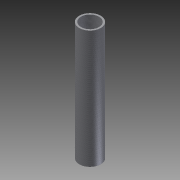
# Autodesk Inventor part: Pusher.Spring(open)
Saved by Autodesk Inventor 2011 (Build 150239000, 239)
## iProperties
Created: 2011-04-01
Part Number: Pusher.Spring(open)
Document SubType Name: Modeling
Designer: Rob
Density: 1 g/cm^3
Author: Rob
Autodesk Inventor part; units mm, degrees
ref_plane "YZ Plane" through (0, 0, 0) normal (1, 0, 0) x (0, 1, 0)
ref_plane "XZ Plane" through (0, 0, 0) normal (0, 1, 0) x (-1, 0, 0)
ref_plane "XY Plane" through (0, 0, 0) normal (0, 0, 1) x (1, 0, 0)
sketch "Sketch1" plane through (0, 0, 0) normal (0, 0, 1) x (1, 0, 0)
  circle A0 centre (0, 0) radius 3.175
  circle A1 centre (0, 0) radius 2.667
  dimension "d0" = 6.35
  dimension "d9" = 5.334
  constraints: 2 centre point, 2 coincident
  measures "d0" diameter of A0
  measures "d9" diameter of A1
coil "Coil2" sketch "Sketch1" operation add axis through (0, 0, -10) along (0, 0, 1) pitch 1.0272 turns 34 hand right
body "Solid2"
